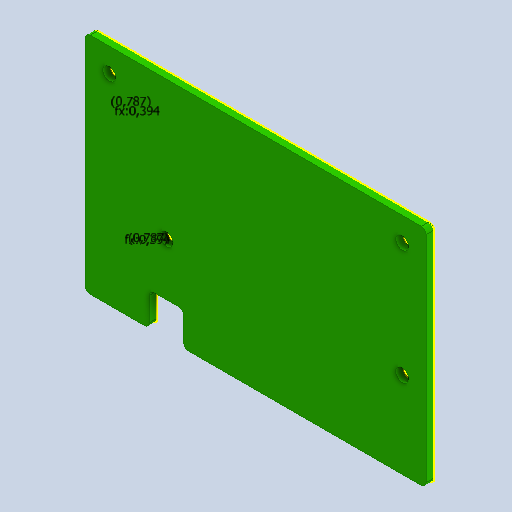
# Autodesk Inventor part: IO_HEADER_PCB
Saved by Autodesk Inventor 2022 (Build 260153000, 153)
## iProperties
Created: 2020-06-15
Part Number: IO_HEADER_PCB
Material: Generic
Document SubType Name: Modeling
Designer: Viktor Lindström
Density: 1 g/cm^3
Appearance: Default
Author: Viktor Lindström
Autodesk Inventor part; units mm, degrees
ref_plane "YZ Plane" through (0, 0, 0) normal (1, 0, 0) x (0, 1, 0)
ref_plane "XZ Plane" through (0, 0, 0) normal (0, 1, 0) x (-1, 0, 0)
ref_plane "XY Plane" through (0, 0, 0) normal (0, 0, 1) x (1, 0, 0)
sketch "Sketch1" plane through (0, 0, 0) normal (0, 0, 1) x (1, 0, 0)
  line L0 (-35.7, -23.5) -> (35.7, -23.5)
  line L1 (35.7, -23.5) -> (35.7, 23.5)
  line L2 (35.7, 23.5) -> (-35.7, 23.5)
  line L3 (-35.7, 23.5) -> (-35.7, -23.5)
  line L4 (-35.7, -23.5) -> (35.7, 23.5) construction
  line L5 (35.7, -23.5) -> (-35.7, 23.5) construction
  point P0 (0, 0)
  dimension "d0" = 47
  dimension "d1" = 71.4
  constraints: 12 end point, 2 midpoint, 2 parallel, 1 horizontal, 1 perpendicular
  measures "d0" distance of L2.end L0.start
  measures "d1" distance between parallel lines of L3 L1
extrude "Extrusion1" add sketch "Sketch1" along normal blind 1.6
sketch "Sketch2" plane through (0, 0, 0) normal (0, 0, -1) x (-1, 0, 0)
  line L0 (35.7, -23.5) -> (-35.7, -23.5) projected
  line L1 (35.7, -23.5) -> (-35.7, -23.5) projected
  line L2 (15.1, -23.5) -> (22.3, -23.5)
  line L3 (22.3, -23.5) -> (22.3, -16.5)
  line L4 (22.3, -16.5) -> (15.1, -16.5)
  line L5 (15.1, -16.5) -> (15.1, -23.5)
  line L6 (-35.7, -23.5) -> (-35.7, 23.5) projected
  point P0 (0, 0)
  dimension "d4" = 50.8
  dimension "d5" = 7.2
  dimension "d6" = 7
  constraints: 8 end point, 2 parallel, 1 horizontal, 1 perpendicular, 1 point on line
  measures "d4" distance between parallel lines of L6 L5
  measures "d5" distance between parallel lines of L5 L3
  measures "d6" distance between parallel lines of L4 L0
extrude "Extrusion2" cut sketch "Sketch2" against normal through all
sketch "Sketch3" plane through (0, 0, 0) normal (0, 0, -1) x (-1, 0, 0)
  circle A0 centre (30.7, 18.5) radius 1.375
  circle A1 centre (-30.7, -5.5) radius 1.375
  circle A2 centre (-30.7, 18.5) radius 1.375
  line L0 (35.7, 23.5) -> (35.7, -23.5) projected
  line L1 (-35.7, 23.5) -> (35.7, 23.5) projected
  line L2 (-35.7, -23.5) -> (-35.7, 23.5) projected
  line L3 (15.1, -23.5) -> (-35.7, -23.5) projected
  circle A3 centre (18.7, -5.5) radius 1.375
  line L4 (15.1, -23.5) -> (15.1, -16.5) projected
  line L5 (22.3, -16.5) -> (22.3, -23.5) projected
  point P0 (0, 0)
  dimension "d9" = 2.75
  dimension "d10" = 2.75
  dimension "d11" = 2.75
  dimension "d12" = 5
  dimension "d13" = 5
  dimension "d14" = 5
  dimension "d15" = 5
  dimension "d16" = 5
  dimension "d17" = 18
  dimension "d20" = 2.75
  dimension "d21" = 0
  dimension "d22" = 7.2
  dimension "d23" = 3.6
  constraints: 4 centre point
  measures "d9" diameter of A0
  measures "d10" diameter of A2
  measures "d11" diameter of A1
  measures "d12" distance from line of L0 A0.centre
  measures "d13" distance from line of L1 A0.centre
  measures "d14" distance from line of L1 A2.centre
  measures "d15" distance from line of L2 A2.centre
  measures "d16" distance from line of L2 A1.centre
  measures "d17" distance from line of L3 A1.centre
  measures "d20" diameter of A3
  measures "d21" vertical distance of A1.centre A3.centre
  measures "d22" distance between parallel lines of L4 L5
  measures "d23" distance from line of A3.centre L5
extrude "Extrusion3" cut sketch "Sketch3" against normal through all
fillet "Fillet1" radius 1 8 edges at (35.7, 23.5, 0.8) (-35.7, 23.5, 0.8) (-35.7, -23.5, 0.8) (-15.1, -23.5, 0.8) (-22.3, -23.5, 0.8) (-15.1, -16.5, 0.8) (-22.3, -16.5, 0.8) (35.7, -23.5, 0.8)
sketch "PWR_PCBA_OUTLINE" plane through (0, 0, 0) normal (0, 0, -1) x (-1, 0, 0)
  line L0 (16.1, -16.5) -> (21.3, -16.5) projected
  arc A0 (16.1, -16.5) -> (15.1, -17.5) centre (16.1, -17.5) ccw projected
  line L1 (15.1, -22.5) -> (15.1, -17.5) projected
  arc A1 (14.1, -23.5) -> (15.1, -22.5) centre (14.1, -22.5) ccw projected
  line L2 (14.1, -23.5) -> (-34.7, -23.5) projected
  arc A2 (-35.7, -22.5) -> (-34.7, -23.5) centre (-34.7, -22.5) ccw projected
  line L3 (-35.7, -22.5) -> (-35.7, 22.5) projected
  arc A3 (-34.7, 23.5) -> (-35.7, 22.5) centre (-34.7, 22.5) ccw projected
  line L4 (-34.7, 23.5) -> (34.7, 23.5) projected
  arc A4 (35.7, 22.5) -> (34.7, 23.5) centre (34.7, 22.5) ccw projected
  line L5 (35.7, 22.5) -> (35.7, -22.5) projected
  arc A5 (34.7, -23.5) -> (35.7, -22.5) centre (34.7, -22.5) ccw projected
  line L6 (34.7, -23.5) -> (23.3, -23.5) projected
  arc A6 (22.3, -22.5) -> (23.3, -23.5) centre (23.3, -22.5) ccw projected
  line L7 (22.3, -17.5) -> (22.3, -22.5) projected
  arc A7 (22.3, -17.5) -> (21.3, -16.5) centre (21.3, -17.5) ccw projected
  circle A8 centre (12.56, -19.5) radius 0.7937
  circle A9 centre (-33.16, -19.5) radius 0.7938
  line L8 (28.691, 15) -> (37.2, 15)
  line L9 (28.691, -10.908) -> (37.2, -10.908)
  line L10 (28.691, -10.908) -> (28.691, -10.4)
  line L11 (28.691, 14.492) -> (28.691, 15)
  line L12 (27.3702, 13.8697) -> (26.9638, 13.8697)
  line L13 (27.3702, 13.623) -> (27.3702, 13.8697)
  line L14 (27.3702, 13.623) -> (27.3702, 13.329)
  line L15 (27.3702, 13.0823) -> (27.3702, 13.329)
  line L16 (26.9638, 13.0823) -> (27.3702, 13.0823)
  line L17 (26.9638, 13.329) -> (26.9638, 13.0823)
  line L18 (26.9638, 13.329) -> (26.9638, 13.623)
  line L19 (26.9638, 13.8697) -> (26.9638, 13.623)
  line L20 (24.8302, -9.237) -> (24.8302, -9.531)
  line L21 (24.8302, -9.237) -> (24.8302, -8.9903)
  line L22 (24.8302, -8.9903) -> (24.4238, -8.9903)
  line L23 (24.4238, -8.9903) -> (24.4238, -9.237)
  line L24 (24.4238, -9.531) -> (24.4238, -9.237)
  line L25 (24.4238, -9.531) -> (24.4238, -9.7777)
  line L26 (24.4238, -9.7777) -> (24.8302, -9.7777)
  line L27 (24.8302, -9.7777) -> (24.8302, -9.531)
  circle A10 centre (24.627, -9.384) radius 0.2032
  circle A11 centre (27.167, 13.476) radius 0.2032
  circle A12 centre (18.7, -5.5) radius 1.375 projected
  circle A13 centre (30.7, 18.5) radius 1.375 projected
  circle A14 centre (-30.7, 18.5) radius 1.375 projected
  circle A15 centre (-30.7, -5.5) radius 1.375 projected
  circle A16 centre (-33.16, -13.5) radius 0.7938
  circle A17 centre (12.56, -13.5) radius 0.7937
  point P0 (0, 0)
  dimension "d29" = 0.7874
  dimension "d30" = 0.3937
  dimension "d31" = 0.3937
  dimension "d32" = 0.7874
  constraints: 40 end point, 14 vertical, 6 centre point, 6 horizontal, 4 tangent, 30 other
  measures "d29" distance between parallel lines of L22 L26
  measures "d30" distance from line of L26 A10.centre
  measures "d31" distance from line of L16 A11.centre
  measures "d32" distance between parallel lines of L16 L12
equation "\"d10\" = d9"
equation "\"d11\" = d9"
equation "\"d13\" = d12"
equation "\"d14\" = d12"
equation "\"d15\" = d12"
equation "\"d16\" = d12"
equation "\"d20\" = d9"
equation "\"d23\" = 0.5 * d22"
equation "\"d30\" = 0.5 * d29"
equation "\"d31\" = 0.5 * d32"
body "Solid1"
